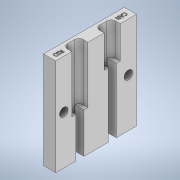
# Autodesk Inventor part: conecter plate
Saved by Autodesk Inventor 2021 (Build 250183000, 183)
## iProperties
Created: 2022-03-10
Part Number: conecter plate
Material: Generic
Document SubType Name: Modeling
Designer: jasmi
Density: 1 g/cm^3
Appearance: Default
Author: jasmi
Autodesk Inventor part; units mm, degrees
ref_plane "YZ Plane" through (0, 0, 0) normal (1, 0, 0) x (0, 1, 0)
ref_plane "XZ Plane" through (0, 0, 0) normal (0, 1, 0) x (-1, 0, 0)
ref_plane "XY Plane" through (0, 0, 0) normal (0, 0, 1) x (1, 0, 0)
sketch "Sketch1" plane through (0, 0, 0) normal (1, 0, 0) x (0, 1, 0)
  line L0 (0, 0) -> (76.2, 0)
  line L1 (76.2, 0) -> (76.2, 63.5)
  line L2 (76.2, 63.5) -> (0, 63.5)
  line L3 (0, 63.5) -> (0, 0)
  dimension "d0" = 63.5
  dimension "d1" = 76.2
  constraints: 8 end point, 2 parallel, 1 horizontal, 1 perpendicular
  measures "d0" distance between parallel lines of L2 L0
  measures "d1" distance of L1.end L2.end
extrude "Extrusion1" add sketch "Sketch1" along normal blind 9.525
sketch "Sketch2" plane through (9.525, 0, 0) normal (1, 0, 0) x (0, 0, -1)
  line L0 (0, 76.2) -> (-63.5, 76.2) projected
  line L1 (-50.8, 76.2) -> (-38.1, 76.2)
  line L2 (-38.1, 76.2) -> (-38.1, 31.75)
  line L3 (-50.8, 31.75) -> (-50.8, 76.2)
  line L4 (-25.4, 76.2) -> (-12.7, 76.2)
  line L5 (-12.7, 76.2) -> (-12.7, 50.8)
  line L6 (-25.4, 50.8) -> (-25.4, 76.2)
  line L7 (-63.5, 76.2) -> (-63.5, 0) projected
  line L8 (0, 0) -> (0, 76.2) projected
  line L9 (-63.5, 0) -> (0, 0) projected
  line L10 (-41.275, 31.75) -> (-41.275, 0)
  line L11 (-41.275, 0) -> (-47.625, 0)
  line L12 (-47.625, 0) -> (-47.625, 31.75)
  line L13 (-15.875, 50.8) -> (-15.875, 0)
  line L14 (-15.875, 0) -> (-22.225, 0)
  line L15 (-22.225, 0) -> (-22.225, 50.8)
  line L16 (-12.7, 50.8) -> (-15.875, 50.8)
  line L17 (-22.225, 50.8) -> (-25.4, 50.8)
  line L18 (-38.1, 31.75) -> (-41.275, 31.75)
  line L19 (-47.625, 31.75) -> (-50.8, 31.75)
  point P0 (-44.45, 76.2)
  point P1 (-44.45, 0)
  point P2 (-19.05, 76.2)
  point P3 (-19.05, 0)
  dimension "d4" = 12.7
  dimension "d6" = 12.7
  dimension "d8" = 12.7
  dimension "d9" = 12.7
  dimension "d10" = 6.35
  dimension "d11" = 6.35
  dimension "d12" = 44.45
  constraints: 32 end point, 8 parallel, 4 midpoint, 4 point on line, 2 horizontal, 2 perpendicular, 2 vertical alignment
  measures "d4" distance between parallel lines of L3 L2
  measures "d6" distance between parallel lines of L6 L5
  measures "d8" distance between parallel lines of L7 L3
  measures "d9" distance between parallel lines of L8 L5
  measures "d10" distance between parallel lines of L12 L10
  measures "d11" distance between parallel lines of L15 L13
  measures "d12" distance from line of L10.start L0
extrude "Extrusion2" cut sketch "Sketch2" against normal blind 7.112 contours L5 L16 L13 L9 L15 L17 L6 L0 | L2 L18 L10 L9 L12 L19 L3 L0
fillet "Fillet1" radius 3.556 5 edges at (2.413, 53.975, 38.1) (2.413, 53.975, 50.8) (2.413, 63.5, 25.4) (2.413, 63.5, 12.7) (2.413, 25.4, 15.875)
sketch "Sketch3" plane through (9.525, 0, 0) normal (1, 0, 0) x (0, 0, -1)
  line L0 (-15.875, 0) -> (0, 0) projected
  line L1 (0, 0) -> (0, 76.2) projected
  line L2 (-47.625, 0) -> (-47.625, 31.75) projected
  line L3 (-63.5, 0) -> (-47.625, 0) projected
  line L4 (-63.5, 76.2) -> (-63.5, 0) projected
  point P0 (-57.15, 38.1)
  point P1 (-6.35, 38.1)
  dimension "d23" = 38.1
  dimension "d24" = 6.35
  dimension "d26" = 38.1
  dimension "d27" = 6.35
  measures "d23" distance from line of point (-6.35, 38.1) L0
  measures "d24" distance from line of L1 point (-6.35, 38.1)
  measures "d26" distance from line of point (-57.15, 38.1) L3
  measures "d27" distance from line of point (-57.15, 38.1) L4
hole "Hole1" at (9.525, 38.1, 57.15) at (9.525, 38.1, 6.35) direction (-1, 0, 0) diameter 6.7469 end through all
sketch "Sketch4" plane through (0, 76.2, 63.5) normal (0, 1, 0) x (1, 0, 0)
  line L0 (6.4802, 60.251) -> (6.4802, 53.7391) construction
  line L1 (6.4802, 53.7391) -> (2.0519, 53.7391) construction
  line L2 (2.0519, 53.7391) -> (2.0519, 60.251) construction
  line L3 (2.0519, 60.251) -> (6.4802, 60.251) construction
  line L4 (7.0359, 9.8782) -> (7.0359, 2.7473) construction
  line L5 (7.0359, 2.7473) -> (3.8595, 2.7473) construction
  line L6 (3.8595, 2.7473) -> (3.8595, 9.8782) construction
  line L7 (3.8595, 9.8782) -> (7.0359, 9.8782) construction
  spline S0 degree 2 poles (3.3235, 58.7517) (3.3235, 59.0481) (3.5236, 59.5495) (3.7237, 59.7323) knots 0 0 0 1 2 2 2
  spline S1 degree 2 poles (3.7237, 59.7323) (3.9213, 59.9151) (4.5141, 60.1152) (4.8994, 60.1152) knots 0 0 0 1 2 2 2
  spline S2 degree 2 poles (4.8994, 60.1152) (5.2823, 60.1152) (5.8504, 59.92) (6.0603, 59.7348) knots 0 0 0 1 2 2 2
  spline S3 degree 2 poles (6.0603, 59.7348) (6.2653, 59.552) (6.4802, 59.053) (6.4802, 58.7443) knots 0 0 0 1 2 2 2
  spline S4 degree 2 poles (6.4802, 58.7443) (6.4802, 58.5912) (6.4358, 58.3219) (6.4012, 58.2083) knots 0 0 0 1 2 2 2
  spline S5 degree 2 poles (6.4012, 58.2083) (6.3691, 58.1095) (6.2777, 57.9045) (6.2233, 57.8032) knots 0 0 0 1 2 2 2
  line L8 (6.2233, 57.8032) -> (5.7343, 57.8032)
  line L9 (5.7343, 57.8032) -> (5.7343, 57.8353)
  spline S6 degree 2 poles (5.7343, 57.8353) (5.7837, 57.8897) (5.922, 58.0576) (5.9887, 58.1787) knots 0 0 0 1 2 2 2
  spline S7 degree 2 poles (5.9887, 58.1787) (6.0529, 58.2948) (6.1344, 58.5689) (6.1344, 58.7468) knots 0 0 0 1 2 2 2
  spline S8 degree 2 poles (6.1344, 58.7468) (6.1344, 58.9419) (5.9739, 59.2902) (5.8207, 59.4211) knots 0 0 0 1 2 2 2
  spline S9 degree 2 poles (5.8207, 59.4211) (5.6651, 59.5495) (5.1933, 59.6928) (4.8994, 59.6928) knots 0 0 0 1 2 2 2
  spline S10 degree 2 poles (4.8994, 59.6928) (4.5857, 59.6928) (4.1337, 59.5421) (3.9781, 59.4112) knots 0 0 0 1 2 2 2
  spline S11 degree 2 poles (3.9781, 59.4112) (3.8274, 59.2828) (3.6743, 58.9394) (3.6743, 58.7468) knots 0 0 0 1 2 2 2
  spline S12 degree 2 poles (3.6743, 58.7468) (3.6743, 58.5714) (3.7607, 58.2725) (3.825, 58.1564) knots 0 0 0 1 2 2 2
  spline S13 degree 2 poles (3.825, 58.1564) (3.8892, 58.0453) (4.0226, 57.8798) (4.0695, 57.8329) knots 0 0 0 1 2 2 2
  line L10 (4.0695, 57.8329) -> (4.0695, 57.8032)
  line L11 (4.0695, 57.8032) -> (3.5854, 57.8032)
  spline S14 degree 2 poles (3.5854, 57.8032) (3.5384, 57.9045) (3.452, 58.0823) (3.4125, 58.2083) knots 0 0 0 1 2 2 2
  spline S15 degree 2 poles (3.4125, 58.2083) (3.368, 58.3417) (3.3235, 58.5689) (3.3235, 58.7517) knots 0 0 0 1 2 2 2
  line L12 (3.3779, 57.7538) -> (6.4259, 56.7263)
  line L13 (6.4259, 56.7263) -> (6.4259, 56.2273)
  line L14 (6.4259, 56.2273) -> (3.3779, 55.1998)
  line L15 (3.3779, 55.1998) -> (3.3779, 55.6271)
  line L16 (3.3779, 55.6271) -> (4.23, 55.9038)
  line L17 (4.23, 55.9038) -> (4.23, 57.0672)
  line L18 (4.23, 57.0672) -> (3.3779, 57.3438)
  line L19 (3.3779, 57.3438) -> (3.3779, 57.7538)
  line L20 (4.5758, 56.0149) -> (6.0109, 56.4867)
  line L21 (6.0109, 56.4867) -> (4.5758, 56.956)
  line L22 (4.5758, 56.956) -> (4.5758, 56.0149)
  line L23 (3.3779, 52.7298) -> (3.3779, 53.1843)
  line L24 (3.3779, 53.1843) -> (6.006, 54.5329)
  line L25 (6.006, 54.5329) -> (3.3779, 54.5329)
  line L26 (3.3779, 54.5329) -> (3.3779, 54.9108)
  line L27 (3.3779, 54.9108) -> (6.4259, 54.9108)
  line L28 (6.4259, 54.9108) -> (6.4259, 54.3353)
  line L29 (6.4259, 54.3353) -> (4.0127, 53.1077)
  line L30 (4.0127, 53.1077) -> (6.4259, 53.1077)
  line L31 (6.4259, 53.1077) -> (6.4259, 52.7298)
  line L32 (6.4259, 52.7298) -> (3.3779, 52.7298)
  line L33 (3.9237, 7.2106) -> (3.9237, 7.7367)
  line L34 (3.9237, 7.7367) -> (5.1364, 8.7)
  line L35 (5.1364, 8.7) -> (5.1364, 9.1644)
  line L36 (5.1364, 9.1644) -> (3.9237, 9.1644)
  line L37 (3.9237, 9.1644) -> (3.9237, 9.5694)
  line L38 (3.9237, 9.5694) -> (6.9717, 9.5694)
  line L39 (6.9717, 9.5694) -> (6.9717, 8.784)
  spline S16 degree 2 poles (6.9717, 8.784) (6.9717, 8.5222) (6.9149, 8.1689) (6.8111, 8.0084) knots 0 0 0 1 2 2 2
  spline S17 degree 2 poles (6.8111, 8.0084) (6.7074, 7.8478) (6.3838, 7.6626) (6.1442, 7.6626) knots 0 0 0 1 2 2 2
  spline S18 degree 2 poles (6.1442, 7.6626) (5.8108, 7.6626) (5.3588, 8.0035) (5.2501, 8.2949) knots 0 0 0 1 2 2 2
  line L40 (5.2501, 8.2949) -> (3.9237, 7.2106)
  spline S19 degree 2 poles (6.1121, 8.085) (6.2455, 8.085) (6.4505, 8.1788) (6.5172, 8.2776) knots 0 0 0 1 2 2 2
  spline S20 degree 2 poles (6.5172, 8.2776) (6.574, 8.3641) (6.6209, 8.5938) (6.6209, 8.7617) knots 0 0 0 1 2 2 2
  line L41 (6.6209, 8.7617) -> (6.6209, 9.1644)
  line L42 (6.6209, 9.1644) -> (5.4748, 9.1644)
  line L43 (5.4748, 9.1644) -> (5.4748, 8.8087)
  spline S21 degree 2 poles (5.4748, 8.8087) (5.4748, 8.6333) (5.5366, 8.3542) (5.6329, 8.2579) knots 0 0 0 1 2 2 2
  spline S22 degree 2 poles (5.6329, 8.2579) (5.7169, 8.1689) (5.954, 8.085) (6.1121, 8.085) knots 0 0 0 1 2 2 2
  line L44 (3.9237, 5.9064) -> (3.9237, 7.0871)
  line L45 (3.9237, 7.0871) -> (4.2349, 7.0871)
  line L46 (4.2349, 7.0871) -> (4.2349, 6.6993)
  line L47 (4.2349, 6.6993) -> (6.6604, 6.6993)
  line L48 (6.6604, 6.6993) -> (6.6604, 7.0871)
  line L49 (6.6604, 7.0871) -> (6.9717, 7.0871)
  line L50 (6.9717, 7.0871) -> (6.9717, 5.9064)
  line L51 (6.9717, 5.9064) -> (6.6604, 5.9064)
  line L52 (6.6604, 5.9064) -> (6.6604, 6.2942)
  line L53 (6.6604, 6.2942) -> (4.2349, 6.2942)
  line L54 (4.2349, 6.2942) -> (4.2349, 5.9064)
  line L55 (4.2349, 5.9064) -> (3.9237, 5.9064)
  spline S23 degree 2 poles (6.6234, 3.2487) (6.4209, 3.0758) (5.8281, 2.8831) (5.4477, 2.8831) knots 0 0 0 1 2 2 2
  spline S24 degree 2 poles (5.4477, 2.8831) (5.0772, 2.8831) (4.477, 3.0708) (4.2744, 3.2487) knots 0 0 0 1 2 2 2
  spline S25 degree 2 poles (4.2744, 3.2487) (4.062, 3.4364) (3.8595, 3.9329) (3.8595, 4.2317) knots 0 0 0 1 2 2 2
  spline S26 degree 2 poles (3.8595, 4.2317) (3.8595, 4.5405) (4.0694, 5.0345) (4.2744, 5.2148) knots 0 0 0 1 2 2 2
  spline S27 degree 2 poles (4.2744, 5.2148) (4.477, 5.3902) (5.0722, 5.5779) (5.4477, 5.5779) knots 0 0 0 1 2 2 2
  spline S28 degree 2 poles (5.4477, 5.5779) (5.8305, 5.5779) (6.4134, 5.3877) (6.6234, 5.2123) knots 0 0 0 1 2 2 2
  spline S29 degree 2 poles (6.6234, 5.2123) (6.8259, 5.0345) (7.0359, 4.538) (7.0359, 4.2317) knots 0 0 0 1 2 2 2
  spline S30 degree 2 poles (7.0359, 4.2317) (7.0359, 3.9205) (6.8185, 3.4216) (6.6234, 3.2487) knots 0 0 0 1 2 2 2
  spline S31 degree 2 poles (5.4477, 3.3055) (5.749, 3.3055) (6.2158, 3.4364) (6.369, 3.555) knots 0 0 0 1 2 2 2
  spline S32 degree 2 poles (6.369, 3.555) (6.5271, 3.676) (6.6851, 4.0168) (6.6851, 4.2293) knots 0 0 0 1 2 2 2
  spline S33 degree 2 poles (6.6851, 4.2293) (6.6851, 4.4491) (6.532, 4.7801) (6.369, 4.9061) knots 0 0 0 1 2 2 2
  spline S34 degree 2 poles (6.369, 4.9061) (6.2134, 5.0271) (5.7441, 5.1555) (5.4477, 5.1555) knots 0 0 0 1 2 2 2
  spline S35 degree 2 poles (5.4477, 5.1555) (4.8475, 5.1555) (4.2102, 4.6516) (4.2102, 4.2293) knots 0 0 0 1 2 2 2
  spline S36 degree 2 poles (4.2102, 4.2293) (4.2102, 3.8069) (4.8475, 3.3055) (5.4477, 3.3055) knots 0 0 0 1 2 2 2
  point P0 (0, 63.5)
  point P1 (4.7625, 56.0563)
  point P2 (6.0205, 6.6695)
  constraints: 4 other
extrude "Extrusion3" cut sketch "Sketch4" against normal blind 1.27
sketch "Sketch5" plane through (0, 0, 0) normal (-1, 0, 0) x (0, 0, 1)
  circle A0 centre (6.35, 38.1) radius 3.3734 projected
  line L0 (12.319, 41.5462) -> (12.319, 34.6538)
  line L1 (12.319, 34.6538) -> (6.35, 31.2076)
  line L2 (6.35, 31.2076) -> (0.381, 34.6538)
  line L3 (0.381, 34.6538) -> (0.381, 41.5462)
  line L4 (0.381, 41.5462) -> (6.35, 44.9924)
  line L5 (6.35, 44.9924) -> (12.319, 41.5462)
  line L6 (51.181, 41.5462) -> (57.15, 44.9924)
  line L7 (57.15, 44.9924) -> (63.119, 41.5462)
  line L8 (63.119, 41.5462) -> (63.119, 34.6538)
  line L9 (63.119, 34.6538) -> (57.15, 31.2076)
  line L10 (57.15, 31.2076) -> (51.181, 34.6538)
  line L11 (51.181, 34.6538) -> (51.181, 41.5462)
  line L12 (0, 0) -> (0, 76.2) projected
  line L13 (63.5, 76.2) -> (63.5, 0) projected
  point P0 (57.15, 38.1)
  dimension "d34" = 11.938
  dimension "d35" = 11.938
  dimension "d36" = 6.35
  constraints: 24 end point, 2 parallel, 1 coincident, 1 horizontal alignment, 26 other
  measures "d34" distance between parallel lines of L0 L3
  measures "d35" distance between parallel lines of L8 L11
  measures "d36" distance from line of L13 point (57.15, 38.1)
extrude "Extrusion4" cut sketch "Sketch5" against normal blind 4.7625
body "Solid1"
